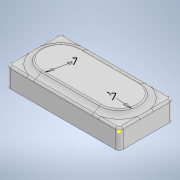
# Autodesk Inventor part: Long Button
Saved by Autodesk Inventor 2021 (Build 250183000, 183)
## iProperties
Created: 2020-05-31
Part Number: Long Button
Material: Generic
Document SubType Name: Modeling
Designer: ameli
Density: 1 g/cm^3
Appearance: Default
Author: ameli
Autodesk Inventor part; units mm, degrees
ref_plane "YZ Plane" through (0, 0, 0) normal (1, 0, 0) x (0, 1, 0)
ref_plane "XZ Plane" through (0, 0, 0) normal (0, 1, 0) x (-1, 0, 0)
ref_plane "XY Plane" through (0, 0, 0) normal (0, 0, 1) x (1, 0, 0)
sketch "Sketch1" plane through (0, 0, 0) normal (0, 1, 0) x (-1, 0, 0)
  line L0 (0, 0) -> (29, 0)
  line L1 (29, 0) -> (29, -14)
  line L2 (29, -14) -> (0, -14)
  line L3 (0, -14) -> (0, 0)
  dimension "d0" = 14
  dimension "d1" = 29
  constraints: 8 end point, 2 parallel, 1 horizontal, 1 perpendicular
  measures "d0" distance of L0.end L1.end
  measures "d1" distance of L1.end L2.end
extrude "Extrusion1" add sketch "Sketch1" along normal blind 5
sketch "Sketch2" plane through (0, 5, 0) normal (0, 1, 0) x (1, 0, 0)
  circle A0 centre (-22, 7) radius 5
  line L0 (-29, 14) -> (-29, 0) projected
  line L1 (0, 14) -> (-29, 14) projected
  circle A1 centre (-7, 7) radius 5
  line L2 (0, 0) -> (0, 14) projected
  line L3 (-22, 12) -> (-7, 12)
  line L4 (-22, 2) -> (-7, 2)
  dimension "d4" = 10
  dimension "d5" = 7
  dimension "d6" = 7
  dimension "d7" = 10
  dimension "d8" = 7
  dimension "d9" = 7
  constraints: 4 end point, 4 point on circle, 2 centre point, 1 parallel, 1 tangent
  measures "d4" diameter of A0
  measures "d5" distance from line of L0 A0.centre
  measures "d6" distance from line of L1 A0.centre
  measures "d7" diameter of A1
  measures "d8" distance from line of L2 A1.centre
  measures "d9" distance from line of L1 A1.centre
extrude "Extrusion2" add sketch "Sketch2" along normal blind 1
fillet "Fillet1" radius 2 4 edges at (-14.5, 5, -2) (-27, 5, -7) (-14.5, 5, -12) (-2, 5, -7)
fillet "Fillet2" radius 0.5 8 edges at (-14.5, 5, 0) (0, 5, -7) (-14.5, 5, -14) (-27, 6, -7) (-14.5, 6, -2) (-2, 6, -7) (-14.5, 6, -12) (-29, 5, -7)
fillet "Fillet3" radius 1 8 edges at (-0.1464, 4.8536, -0.1464) (0, 2.25, 0) (-0.1464, 4.8536, -13.8536) (0, 2.25, -14) (-28.8536, 4.8536, -0.1464) (-29, 2.25, 0) (-28.8536, 4.8536, -13.8536) (-29, 2.25, -14)
shell "Shell1" thickness 1.5 removed faces 1 at (-19, 0, -9.3333)
sketch "Sketch3" plane through (-22, 4.5, -2.7174) normal (0, -1, 0) x (1, 0, 0)
  circle A0 centre (15, -4.2826) radius 3.5
  arc A1 (15, -8.5651) -> (15, 0) centre (15, -4.2826) ccw projected
  circle A2 centre (0, -4.2826) radius 3.5
  arc A3 (0, 0) -> (0, -8.5651) centre (0, -4.2826) ccw projected
  point P0 (22, 2.7174)
  dimension "d16" = 7
  dimension "d17" = 7
  constraints: 2 centre point, 2 concentric
  measures "d16" diameter of A0
  measures "d17" diameter of A2
body "Solid1"
